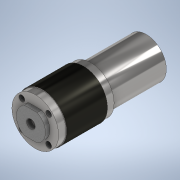
# Autodesk Inventor part: motor_body
Saved by Autodesk Inventor 2020 (Build 240168000, 168)
## iProperties
Created: 2020-07-28
Part Number: motor_body
Material: Steel, Mild
Document SubType Name: Modeling
Designer: Ashiqrahman
Density: 7.85 g/cm^3
Appearance: Semi-Polished
Mass: 434.918 g
Surface Area: 95.2129 cm^2
Volume: 55.4036 cm^3
Author: Ashiqrahman
Autodesk Inventor part; units mm, degrees
sketch "Sketch1" plane through (0, 0, 0) normal (0, 0, 1) x (1, 0, 0)
  circle A0 centre (0, 0) radius 13.8
  dimension "d0" = 27.6
  constraints: 1 centre point, 1 coincident
  measures "d0" diameter of A0
extrude "Extrusion1" add sketch "Sketch1" against normal blind 76
ref_plane "Work Plane1" through (0, 0, -38) normal (0, 0, 1) x (1, 0, 0)
sketch "Sketch2" plane through (0, 0, -38) normal (0, 0, 1) x (1, 0, 0)
  circle A0 centre (0, 0) radius 13.8 projected
  circle A1 centre (0, 0) radius 16
  dimension "d4" = 32
  constraints: 1 centre point, 1 coincident
  measures "d4" diameter of A1
extrude "Extrusion2" add sketch "Sketch2" along normal blind 38
sketch "Sketch3" plane through (0, 0, -76) normal (0, 0, -1) x (-1, 0, 0)
  circle A0 centre (0, 0) radius 5
  dimension "d7" = 10
  constraints: 1 centre point, 1 coincident
  measures "d7" diameter of A0
extrude "Extrusion3" add sketch "Sketch3" along normal blind 2
sketch "Sketch4" plane through (0, 0, 0) normal (0, 0, 1) x (1, 0, 0)
  circle A0 centre (0, 0) radius 5 projected
  circle A1 centre (0, 0) radius 10
  line L0 (-4.3589, -9) -> (4.3589, -9)
  line L1 (4.3589, -9) -> (4.3589, 9)
  line L2 (4.3589, 9) -> (-4.3589, 9)
  line L3 (-4.3589, 9) -> (-4.3589, -9)
  line L4 (-4.3589, -9) -> (4.3589, 9) construction
  line L5 (4.3589, -9) -> (-4.3589, 9) construction
  dimension "d10" = 20
  dimension "d11" = 18
  constraints: 12 end point, 2 midpoint, 2 parallel, 1 coincident, 1 horizontal, 1 perpendicular, 3 other
  measures "d11" distance of L1.end L0.end
extrude "Extrusion4" add sketch "Sketch4" along normal blind 3 contours A0 L1 | A0 L1 A1 | L1 A0 L3 | A0 L3 L2 L1 | L1 L0 L3 A0 | L3 A0 | A0 L3 A1
sketch "Sketch5" plane through (0, 0, 3) normal (0, 0, 1) x (1, 0, 0)
  circle A0 centre (0, 0) radius 3
  dimension "d14" = 6
  constraints: 1 centre point, 1 coincident
  measures "d14" diameter of A0
extrude "Extrusion5" cut sketch "Sketch5" against normal blind 3
sketch "Sketch6" plane through (0, 0, 0) normal (0, 0, 1) x (1, 0, 0)
  circle A0 centre (0, 0) radius 3 projected
  circle A1 centre (0, 0) radius 13
  line L0 (0, 0) -> (9.1924, 9.1924)
  line L1 (0, 0) -> (13, 0) construction
  circle A2 centre (9.1924, 9.1924) radius 2
  dimension "d17" = 26
  dimension "d18" = 45
  dimension "d19" = 4
  constraints: 4 end point, 2 coincident, 1 centre point, 1 equal length, 1 horizontal, 3 other
  measures "d18" angle of L1 L0
  measures "d19" diameter of A2
extrude "Extrusion6" cut sketch "Sketch6" against normal blind 6 contours A2 A1 L0 | L0 A1 A2 | A1 A2 picked at (9.9348, 9.3429)
pattern_circular "Circular Pattern1" count 4 over 360 about axis through (0, 0, -38) along (0, 0, 1) of "Extrusion6"
ref_plane "Work Plane2" through (0, 0, -5) normal (0, 0, 1) x (1, 0, 0)
ref_plane "Work Plane3" through (0, 0, -33) normal (0, 0, -1) x (-1, 0, 0)
sketch "Sketch7" plane through (0, 0, -5) normal (0, 0, 1) x (1, 0, 0)
  circle A0 centre (9.1924, -9.1924) radius 2 projected
  circle A1 centre (-9.1924, -9.1924) radius 2 projected
  circle A2 centre (-9.1924, 9.1924) radius 2 projected
  circle A3 centre (9.1924, 9.1924) radius 2 projected
  line L0 (4.3589, -9) -> (-4.3589, -9) projected
  arc A4 (-4.3589, 9) -> (-4.3589, -9) centre (0, 0) ccw projected
  line L1 (-4.3589, 9) -> (4.3589, 9) projected
  arc A5 (4.3589, -9) -> (4.3589, 9) centre (0, 0) ccw projected
  circle A6 centre (0, 0) radius 16 projected
  circle A7 centre (0, 0) radius 3 projected
  circle A8 centre (0, 0) radius 16.5
  dimension "d27" = 33
  constraints: 1 centre point, 1 coincident
  measures "d27" diameter of A8
extrude "Extrusion7" add sketch "Sketch7" against normal up to surface (28 mm away) contours A8
thread "Thread1" size "M4x0.7" class "6H" standard "ANSI Metric M Profile" length 60
thread "Thread2" size "M4x0.7" class "6H" standard "ANSI Metric M Profile" length 60
thread "Thread3" size "M4x0.7" class "6H" standard "ANSI Metric M Profile" length 60
thread "Thread4" size "M4x0.7" class "6H" standard "ANSI Metric M Profile" length 60
body "Solid1"
